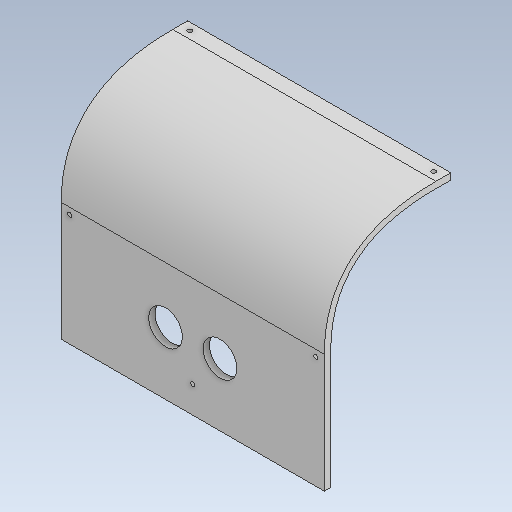
# Autodesk Inventor part: frente recurva
Saved by Autodesk Inventor 2020 (Build 240168000, 168)
## iProperties
Created: 2020-04-24
Part Number: frente recurva
Material: Genérico
Document SubType Name: Modeling
Designer: gi-se
Density: 1 g/cm^3
Appearance: Padrão
Author: gi-se
Autodesk Inventor part; units mm, degrees
ref_plane "YZ Plane" through (0, 0, 0) normal (1, 0, 0) x (0, 1, 0)
ref_plane "XZ Plane" through (0, 0, 0) normal (0, 1, 0) x (-1, 0, 0)
ref_plane "XY Plane" through (0, 0, 0) normal (0, 0, 1) x (1, 0, 0)
sketch "Esboço1" plane through (0, 0, 0) normal (0, 0, 1) x (1, 0, 0)
  line L0 (-21.8, -28.4) -> (-21.8, -58.8) projected
  line L1 (-16.1, -47.2) -> (-23.9, -47.2) projected
  line L2 (-26.1, 49.6356) -> (-29.1, 49.6356) projected
  line L3 (-21.8, -47.2) -> (101.8, -47.2)
  line L4 (101.8, -47.2) -> (101.8, 49.6356)
  line L5 (101.8, 49.6356) -> (-21.8, 49.6356)
  line L6 (-21.8, 49.6356) -> (-21.8, -47.2)
  line L7 (101.8, -28.4) -> (101.8, -58.8) projected
  circle A0 centre (27.2, -17.8) radius 7.95 projected
  circle A1 centre (52.8, -17.8) radius 7.95 projected
  circle A2 centre (40, -34.6) radius 1 projected
  line L8 (-0.0154, 1.5) -> (75.5655, 1.5) projected
  line L9 (75.5655, 1.5) -> (106.1, 1.5) projected
  line L10 (-26.1, 1.5) -> (-0.0154, 1.5) projected
  point P0 (0, 0)
  point P1 (-21.8, 1.5)
  point P2 (101.8, 1.5)
  dimension "d0" = 0
  constraints: 8 end point, 2 parallel, 2 point on line, 1 horizontal, 1 perpendicular
  measures "d0" distance between parallel lines of L7 L4
extrude "Extrusão1" add sketch "Esboço1" along normal blind 3 contours L6 L10 L8 L9 L4 L3 L1 L0
sketch "Esboço2" plane through (101.8, -47.2, 0) normal (1, 0, 0) x (0, 0, -1)
  line L0 (0, 48.7) -> (0, 0)
  line L1 (0, 48.7) -> (-3, 48.7)
  line L2 (-3, 48.7) -> (-3, 55.7)
  line L3 (-3, 55.7) -> (0, 55.7)
  line L4 (0, 55.7) -> (0, 48.7)
  line L5 (16.4, 7.2) -> (16.4, 89.4875)
  line L6 (67.3088, 7.2) -> (16.4, 7.2)
  line L7 (57.4544, 17.0544) -> (67.3088, 7.2)
  arc A0 (56.4, 19.6) -> (57.4544, 17.0544) centre (60, 19.6) ccw
  line L8 (56.4, 35.6) -> (56.4, 19.6)
  arc A1 (63.6, 35.6) -> (56.4, 35.6) centre (60, 35.6) ccw
  line L9 (63.6, 21.0912) -> (63.6, 35.6)
  line L10 (77.4912, 7.2) -> (63.6, 21.0912)
  line L11 (109.9, 7.2) -> (77.4912, 7.2)
  line L12 (109.9, 77.4021) -> (109.9, 7.2)
  line L13 (53.4, 87.3646) -> (109.9, 77.4021)
  line L14 (53.4, 90.3646) -> (53.4, 87.3646)
  line L15 (56.4, 90.3646) -> (53.4, 90.3646)
  line L16 (56.4, 96.8356) -> (56.4, 90.3646)
  line L17 (49.4, 96.8356) -> (56.4, 96.8356)
  spline S0 degree 2 poles (16.4, 89.4875) (28.4788, 96.8356) (49.4, 96.8356) knots 0 0 0 1 1 1
  circle A2 centre (49.1, 41) radius 0.8
  line L18 (0, 55.7) -> (0, 96.8356) construction
  line L19 (0, 96.8356) -> (49.4, 96.8356) construction
  spline S1 degree 2 poles (0, 55.7) (0, 96.8356) (49.4, 96.8356) knots 1 1 1 2 2 2
  line L20 (49.4, 99.8356) -> (56.4, 99.8356)
  line L21 (56.4, 99.8356) -> (56.4, 96.8356)
  line L22 (56.4, 96.8356) -> (49.4, 96.8356)
  line L23 (49.4, 96.8356) -> (49.4, 99.8356)
  spline S2 degree 5 poles (-3, 55.7) (-3.0006, 59.6028) (-2.7317, 63.5042) (-2.1469, 67.3846) (-0.2515, 74.6) (3.2657, 81.1646) (5.3254, 84.0489) (10.316, 89.3567) (16.4783, 93.2583) (19.8737, 94.8743) (27.6563, 97.7143) (35.8292, 99.1582) (40.3418, 99.6246) (44.8718, 99.8357) (49.4, 99.8356) knots 0 0 0 0 0 0 0.249163 0.249163 0.249163 0.472611 0.472611 0.472611 0.710868 0.710868 0.710868 1 1 1 1 1 1
  point P0 (0, 47.2)
  point P1 (16.4, 89.4467)
  dimension "d3" = 7
  constraints: 16 end point, 4 parallel, 3 perpendicular, 2 horizontal, 1 collinear, 6 other
  measures "d3" distance of L1.end L2.end
extrude "Extrusão2" add sketch "Esboço2" against normal blind 123.6 contours L1 L2 L3 L4 | L3 S2 L23 S0 L5 S1 | L20 L21 L17 L23
sketch "Esboço3" plane through (0, 0, 3) normal (0, 0, 1) x (1, 0, 0)
  circle A0 centre (-17.8, 5.5) radius 1 projected
  circle A1 centre (97.8, 5.5) radius 1 projected
  point P0 (0, 0)
extrude "Extrusão3" cut sketch "Esboço3" against normal blind 6
sketch "Esboço4" plane through (101.8, 52.6356, -49.4) normal (0, 1, 0) x (1, 0, 0)
  circle A0 centre (-119.1, 3.5) radius 1 projected
  circle A1 centre (-4.5, 3.5) radius 1 projected
  point P0 (-101.8, -49.4)
extrude "Extrusão4" cut sketch "Esboço4" against normal blind 6
